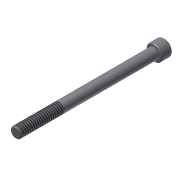
# Autodesk Inventor part: 14-20 x750
Saved by Autodesk Inventor 2013 (Build 170138000, 138)
## iProperties
Created: 2011-07-22
Part Number: 14-20 x750
Material: Steel
Document SubType Name: Modeling
Designer: Dan Niemitalo
Mass: 4.73589 g
Surface Area: 4.43369 cm^2
Volume: 0.603299 cm^3
Density: 7.85 g/cm^3
Author: Dan Niemitalo
Autodesk Inventor part; units mm, degrees
ref_plane "YZ Plane" through (0, 0, 0) normal (1, 0, 0) x (0, 1, 0)
ref_plane "XZ Plane" through (0, 0, 0) normal (0, 1, 0) x (-1, 0, 0)
ref_plane "XY Plane" through (0, 0, 0) normal (0, 0, 1) x (1, 0, 0)
sketch "Sketch1" plane through (0, 0, 0) normal (0, 0, 1) x (1, 0, 0)
  circle A0 centre (0, 0) radius 3.175
  dimension "d0" = 6.35
  constraints: 1 centre point, 1 coincident
  measures "d0" diameter of A0
extrude "Extrusion1" add sketch "Sketch1" along normal blind 82.55
sketch "Sketch2" plane through (0, 0, 0) normal (0, 0, -1) x (-1, 0, 0)
  circle A0 centre (0, 0) radius 3.175 projected
  circle A1 centre (0, 0) radius 4.7625
  dimension "d3" = 9.525
  constraints: 1 centre point, 1 coincident
  measures "d3" diameter of A1
extrude "Extrusion2" add sketch "Sketch2" along normal blind 6.35 contours A0 | A1
sketch "Sketch3" plane through (0, 0, -6.35) normal (0, 0, -1) x (-1, 0, 0)
  circle A0 centre (0, 0) radius 4.7625 projected
  line L0 (-1.3748, 2.3812) -> (1.3748, 2.3813)
  line L1 (1.3748, 2.3813) -> (2.7496, 0)
  line L2 (2.7496, 0) -> (1.3748, -2.3812)
  line L3 (1.3748, -2.3812) -> (-1.3748, -2.3812)
  line L4 (-1.3748, -2.3812) -> (-2.7496, 0)
  line L5 (-2.7496, 0) -> (-1.3748, 2.3812)
  dimension "d6" = 4.7625
  constraints: 12 end point, 1 coincident, 1 horizontal, 13 other
  measures "d6" distance between parallel lines of L3 L0
extrude "Extrusion3" cut sketch "Sketch3" against normal blind 3.175 contours L0 L1 L2 L3 L4 L5
chamfer "Chamfer1" distance 0.508 angle 45 3 edges at (-3.175, 0, 82.55) (4.7625, 0, 0) (4.7625, 0, -6.35)
thread "Thread1" size "1/4-20 UNC" class "2A" standard "ANSI Unified Screw Threads" length 25.4
body "Solid1"
